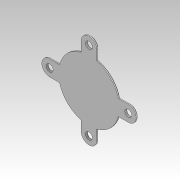
# Autodesk Inventor part: PlatformBracket
Saved by Autodesk Inventor 2020 (Build 240168000, 168)
## iProperties
Created: 2021-08-24
Part Number: PlatformBracket
Material: Generic
Document SubType Name: Modeling
Designer: DDeGo
Density: 1 g/cm^3
Appearance: Default
Author: DDeGo
Autodesk Inventor part; units mm, degrees
ref_plane "YZ Plane" through (0, 0, 0) normal (1, 0, 0) x (0, 1, 0)
ref_plane "XZ Plane" through (0, 0, 0) normal (0, 1, 0) x (-1, 0, 0)
ref_plane "XY Plane" through (0, 0, 0) normal (0, 0, 1) x (1, 0, 0)
sketch "Sketch1" plane through (0, 0, 0) normal (0, 0, 1) x (1, 0, 0)
  circle A0 centre (0, 0) radius 15.5
  line L0 (-20, 0) -> (20, 0) construction
  line L1 (-20, -4) -> (20, -4)
  line L2 (20, 4) -> (-20, 4)
  arc A1 (-20, 4) -> (-20, -4) centre (-20, 0) ccw
  arc A2 (20, -4) -> (20, 4) centre (20, 0) ccw
  line L3 (0, -20) -> (0, 20) construction
  line L4 (4, -20) -> (4, 20)
  line L5 (-4, 20) -> (-4, -20)
  arc A3 (-4, -20) -> (4, -20) centre (0, -20) ccw
  arc A4 (4, 20) -> (-4, 20) centre (0, 20) ccw
  circle A5 centre (-20, 0) radius 1.75
  circle A6 centre (0, 20) radius 1.75
  circle A7 centre (20, 0) radius 1.75
  circle A8 centre (0, -20) radius 1.75
  point P0 (4, -14.975)
  point P1 (14.975, -4)
  point P2 (14.975, 4)
  point P3 (4, 14.975)
  point P4 (-4, 14.975)
  point P5 (-14.975, 4)
  point P6 (-14.975, -4)
  point P7 (-4, -14.975)
  dimension "d0" = 40
  dimension "d1" = 40
  dimension "d2" = 4
  dimension "d3" = 4
  dimension "d4" = 31
  dimension "d5" = 3.5
  constraints: 16 end point, 9 centre point, 8 point on circle, 8 tangent, 5 coincident, 3 equal radius, 2 midpoint, 2 parallel, 1 horizontal, 1 perpendicular
  measures "d0" distance of L0.start L0.end
  measures "d1" distance of L3.start L3.end
  measures "d2" radius of A2
  measures "d3" radius of A3
  measures "d4" diameter of A0
  measures "d5" diameter of A5
extrude "Extrusion1" add sketch "Sketch1" along normal blind 1
chamfer "Chamfer1" distance 0.5 angle 45 16 edges at (-10.9602, -10.9602, 0) (-4, -17.4875, 0) (0, -24, 0) (4, -17.4875, 0) (10.9602, -10.9602, 0) (17.4875, -4, 0) (24, 0, 0) (17.4875, 4, 0) (10.9602, 10.9602, 0) (4, 17.4875, 0) (0, 24, 0) (-4, 17.4875, 0) (-10.9602, 10.9602, 0) (-17.4875, 4, 0) (-24, 0, 0) (-17.4875, -4, 0)
body "Solid1"
